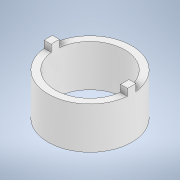
# Autodesk Inventor part: upperBase1
Saved by Autodesk Inventor 2021 (Build 250183000, 183)
## iProperties
Created: 2021-01-06
Part Number: upperBase1
Material: Generic
Document SubType Name: Modeling
Designer: awitc
Density: 1 g/cm^3
Appearance: Smooth - White
Author: awitc
Autodesk Inventor part; units mm, degrees
ref_plane "YZ Plane" through (0, 0, 0) normal (1, 0, 0) x (0, 1, 0)
ref_plane "XZ Plane" through (0, 0, 0) normal (0, 1, 0) x (-1, 0, 0)
ref_plane "XY Plane" through (0, 0, 0) normal (0, 0, 1) x (1, 0, 0)
sketch "Sketch1" plane through (0, 0, 0) normal (0, 1, 0) x (-1, 0, 0)
  line L0 (0, 0) -> (50, 0) construction
  line L1 (0, 0) -> (50, 0) construction
  line L2 (0, 0) -> (-36, 0)
  circle A0 centre (0, 0) radius 25
  line L3 (-60, -10) -> (-60, 10)
  circle A1 centre (0, 0) radius 61
  point P0 (62.509, -33.0548)
  point P1 (12.6591, 21.558)
  point P2 (24.4148, 5.3777)
  point P3 (24.4148, -5.3777)
  point P4 (-22.9129, 10)
  point P5 (-22.9129, -10)
  point P6 (12.6591, -21.558)
  dimension "d2" = 36
  dimension "d3" = 50
  dimension "d26" = 122
  constraints: 8 end point, 6 point on circle, 3 horizontal, 2 centre point, 2 coincident
  measures "d2" distance of L2.start L2.end
  measures "d3" diameter of A0
  measures "d26" diameter of A1
extrude "Extrusion1" add sketch "Sketch1" along normal blind 5 contours A0 | A1
sketch "Sketch2" plane through (0, 5, 0) normal (0, 1, 0) x (1, 0, 0)
  circle A0 centre (0, 0) radius 20
  dimension "d6" = 40
  constraints: 1 centre point, 1 coincident
  measures "d6" diameter of A0
extrude "Extrusion2" cut sketch "Sketch2" against normal up to next
sketch "Sketch3" plane through (0, 5, 0) normal (0, 1, 0) x (1, 0, 0)
  line L0 (22.1416, 4) -> (20.8701, 4)
  line L1 (22.1416, -4) -> (20.8701, -4)
  line L2 (24.6779, 4) -> (22.1416, 4)
  line L3 (24.6779, -4) -> (22.1416, -4)
  line L4 (-15.5618, -16.2506) -> (-14.5332, -15.5032)
  line L5 (-15.5618, 16.2506) -> (-14.5332, 15.5032)
  line L6 (-20.2641, -9.7784) -> (-19.2354, -9.0311)
  line L7 (-17.6137, -17.7414) -> (-15.5618, -16.2506)
  line L8 (-22.316, -11.2693) -> (-20.2641, -9.7784)
  line L9 (-20.2641, 9.7784) -> (-19.2354, 9.0311)
  line L10 (-17.6137, 17.7414) -> (-15.5618, 16.2506)
  line L11 (-22.316, 11.2693) -> (-20.2641, 9.7784)
  line L12 (-23.5374, 22.0452) -> (-13.679, 22.0452) construction
  arc A0 (-17.6137, -17.7414) -> (24.6779, -4) centre (0, 0) ccw
  arc A1 (24.6779, 4) -> (-17.6137, 17.7414) centre (0, 0) ccw
  arc A2 (-22.316, 11.2693) -> (-22.316, -11.2693) centre (0, 0) ccw
  line L13 (20.8701, 4) -> (15.8701, 4)
  line L14 (15.8701, 4) -> (15.8701, -4)
  line L15 (15.8701, -4) -> (20.8701, -4)
  line L16 (-14.5332, 15.5032) -> (-10.4881, 12.5643)
  line L17 (-10.4881, 12.5643) -> (-15.1903, 6.0922)
  line L18 (-15.1903, 6.0922) -> (-19.2354, 9.0311)
  line L19 (-19.2354, -9.0311) -> (-15.1903, -6.0922)
  line L20 (-15.1903, -6.0922) -> (-10.4881, -12.5643)
  line L21 (-10.4881, -12.5643) -> (-14.5332, -15.5032)
  circle A3 centre (-22.5, 0) radius 1.5
  circle A4 centre (0, 22.5) radius 1.5
  circle A5 centre (18.2029, 13.2252) radius 1.5
  circle A6 centre (18.2029, -13.2252) radius 1.5
  circle A7 centre (0, -22.5) radius 1.5
  circle A8 centre (0, 0) radius 4
  line L22 (0, 0) -> (8, 0)
  line L23 (8, 0) -> (8, 7.5)
  line L24 (8, 0) -> (8, -7.5)
  circle A9 centre (8, -7.5) radius 2.5
  circle A10 centre (8, 7.5) radius 2.5
  point P0 (-23.5374, -22.0452)
  point P1 (-28.2397, -15.5731)
  dimension "d9" = 36
  dimension "d10" = 5
  dimension "d11" = 5
  dimension "d12" = 3
  dimension "d13" = 3
  dimension "d14" = 3
  dimension "d15" = 3
  dimension "d16" = 3
  dimension "d17" = 8
  dimension "d18" = 8
  dimension "d19" = 7.5
  dimension "d20" = 7.5
  dimension "d21" = 5
  dimension "d22" = 5
  constraints: 50 end point, 11 centre point, 6 point on circle, 5 parallel, 4 coincident, 4 horizontal, 4 perpendicular, 2 vertical
  measures "d9" angle of L10 L12
  measures "d10" distance of L15.end L15.start
  measures "d11" distance of L16.start L17.start
  measures "d12" diameter of A3
  measures "d13" diameter of A4
  measures "d14" diameter of A5
  measures "d15" diameter of A6
  measures "d16" diameter of A7
  measures "d17" diameter of A8
  measures "d18" distance of L22.start L24.start
  measures "d19" distance of L24.start L23.end
  measures "d20" distance of L24.start L24.end
  measures "d21" diameter of A9
  measures "d22" diameter of A10
extrude "Extrusion3" cut sketch "Sketch3" against normal up to next contours A3 | A4 | A5 | A6 | A7
sketch "Sketch5" plane through (0, 5, 0) normal (0, 1, 0) x (1, 0, 0)
  line L0 (0, 0) -> (37.5601, 0) construction
  circle A0 centre (0, 0) radius 25
  line L1 (0, 0) -> (15.7675, -27.31)
  line L2 (0, 0) -> (31.5349, 0) construction
  line L3 (0, 0) -> (19.8269, 34.3411)
  line L4 (0, 0) -> (39.6537, 0) construction
  line L5 (12.5, 21.6506) -> (15, 25.9808)
  line L6 (12.5, -21.6506) -> (15, -25.9808)
  line L7 (15, -25.9808) -> (27.9904, -18.4808)
  line L8 (27.9904, -18.4808) -> (34.9904, -30.6051)
  line L9 (34.9904, -30.6051) -> (22, -38.1051)
  line L10 (22, -38.1051) -> (15, -25.9808)
  line L11 (22, -38.1051) -> (15, -25.9808)
  line L12 (15, -25.9808) -> (2.0096, -33.4808)
  line L13 (2.0096, -33.4808) -> (9.0096, -45.6051)
  line L14 (9.0096, -45.6051) -> (22, -38.1051)
  line L15 (15, 25.9808) -> (2.0096, 33.4808)
  line L16 (2.0096, 33.4808) -> (9.0096, 45.6051)
  line L17 (9.0096, 45.6051) -> (22, 38.1051)
  line L18 (22, 38.1051) -> (15, 25.9808)
  line L19 (22, 38.1051) -> (15, 25.9808)
  line L20 (15, 25.9808) -> (27.9904, 18.4808)
  line L21 (27.9904, 18.4808) -> (34.9904, 30.6051)
  line L22 (34.9904, 30.6051) -> (22, 38.1051)
  dimension "d41" = 50
  dimension "d47" = 60
  dimension "d48" = 60
  dimension "d49" = 5
  dimension "d50" = 5
  dimension "d51" = 15
  dimension "d52" = 14
  dimension "d53" = 15
  dimension "d54" = 15
  dimension "d55" = 14
  dimension "d56" = 15
  constraints: 46 end point, 11 equal length, 6 perpendicular, 4 point on line, 3 horizontal, 2 point on circle, 1 centre point, 1 coincident
  measures "d41" diameter of A0
  measures "d47" angle of L1 L2
  measures "d48" angle of L4 L3
  measures "d49" distance of L5.start L5.end
  measures "d50" distance of L6.start L6.end
  measures "d51" distance of L6.end L7.end
  measures "d52" distance of L7.end L8.end
  measures "d53" distance of L12.end L6.end
  measures "d54" distance of L5.end L15.end
  measures "d55" distance of L15.end L16.end
  measures "d56" distance of L20.end L5.end
extrude "Extrusion5" cut sketch "Sketch5" against normal up to next contours L7 L8 L9 L10 L1 | L1 L10 L14 L13 L12 | L15 L16 L17 L18 L3 | L3 L18 L22 L21 L20
sketch "Sketch6" plane through (0, 0, 0) normal (0, -1, 0) x (1, 0, 0)
  circle A0 centre (0, 0) radius 25
  circle A1 centre (0, 0) radius 28.75
  circle A2 centre (0, 0) radius 30
  dimension "d57" = 50
  dimension "d58" = 57.5
  constraints: 3 centre point, 3 coincident
  measures "d57" diameter of A0
  measures "d58" diameter of A1
extrude "Extrusion6" add sketch "Sketch6" along normal blind 30 contours A1 | A2
sketch "Sketch7" plane through (0, -30, 0) normal (0, -1, 0) x (1, 0, 0)
  circle A0 centre (26.875, 0) radius 1.5
  circle A1 centre (0, -26.875) radius 1.5
  circle A2 centre (-26.875, 0) radius 1.5
  circle A3 centre (0, 26.875) radius 1.5
  circle A4 centre (19.0035, 19.0035) radius 1.5
  circle A5 centre (19.0035, -19.0035) radius 1.5
  circle A6 centre (-19.0035, -19.0035) radius 1.5
  circle A7 centre (-19.0035, 19.0035) radius 1.5
  dimension "d62" = 3
  dimension "d63" = 3
  dimension "d64" = 3
  dimension "d65" = 3
  dimension "d67" = 3
  dimension "d68" = 3
  dimension "d69" = 3
  dimension "d70" = 3
  constraints: 8 centre point
  measures "d62" diameter of A0
  measures "d63" diameter of A1
  measures "d64" diameter of A2
  measures "d65" diameter of A3
  measures "d67" diameter of A4
  measures "d68" diameter of A5
  measures "d69" diameter of A6
  measures "d70" diameter of A7
extrude "Extrusion7" cut sketch "Sketch7" against normal blind 10
sketch "Sketch8" plane through (0, 0, 0) normal (0, -1, 0) x (1, 0, 0)
  line L0 (-37.9479, -22.6265) -> (-41.4746, -17.7724)
  line L1 (-47.9467, -22.4747) -> (-44.42, -27.3288)
  line L2 (-31.2231, -27.6292) -> (-27.6611, -32.4577)
  circle A0 centre (-42.9473, -22.5506) radius 1.5
  circle A1 centre (-26.2405, -27.6816) radius 1.5
  line L3 (-29.7189, 33.9527) -> (-36.191, 38.655)
  line L4 (-39.7177, 33.8009) -> (-33.2456, 29.0986)
  line L5 (-29.4532, 16.4547) -> (-35.9253, 21.157)
  line L6 (41.5, 10) -> (33.5, 10)
  line L7 (33.5, 4) -> (41.5, 4)
  line L8 (44, -10) -> (52, -10)
  circle A2 centre (48, -7) radius 1.5
  circle A3 centre (37.5, 7) radius 1.5
  circle A4 centre (-34.7183, 33.8768) radius 1.5
  circle A5 centre (-34.4526, 16.3788) radius 1.5
  point P0 (0, 0)
  point P1 (0, 0)
  point P2 (-32.9799, 11.6006)
  point P3 (44, -4)
  dimension "d73" = 3
  dimension "d74" = 3
  dimension "d75" = 3
  dimension "d76" = 3
  dimension "d77" = 3
  constraints: 18 end point, 6 centre point
  measures "d73" diameter of A0
  measures "d74" diameter of A1
  measures "d75" diameter of A2
  measures "d76" diameter of A3
  measures "d77" diameter of A5
extrude "Extrusion8" cut sketch "Sketch8" against normal blind 5
sketch "Sketch9" plane through (0, 5, 0) normal (0, 1, 0) x (1, 0, 0)
  line L0 (2.0096, -33.4808) -> (27.9904, -18.4808) projected
  line L1 (9.0096, -45.6051) -> (2.0096, -33.4808)
  line L2 (2.0096, -33.4808) -> (-0.5885, -34.9808)
  line L3 (-0.5885, -34.9808) -> (6.4115, -47.1051)
  line L4 (6.4115, -47.1051) -> (9.0096, -45.6051)
  line L5 (2.0096, 33.4808) -> (9.0096, 45.6051) projected
  line L6 (2.0096, 33.4808) -> (9.0096, 45.6051)
  line L7 (9.0096, 45.6051) -> (6.4115, 47.1051)
  line L8 (6.4115, 47.1051) -> (-0.5885, 34.9808)
  line L9 (-0.5885, 34.9808) -> (2.0096, 33.4808)
  point P0 (0, 0)
  dimension "d80" = 3
  dimension "d81" = 3
  constraints: 16 end point, 4 parallel, 3 perpendicular, 1 point on line
  measures "d80" distance of L2.end L0.start
  measures "d81" distance of L7.end L6.end
extrude "Extrusion9" cut sketch "Sketch9" against normal blind 10
sketch "Sketch10" plane through (0, 0, 0) normal (0, -1, 0) x (1, 0, 0)
  line L0 (6.4115, 47.1051) -> (-9.1769, 56.1051)
  line L1 (-9.1769, 56.1051) -> (-16.1769, 43.9808)
  line L2 (-16.1769, 43.9808) -> (-0.5885, 34.9808)
  line L3 (-9.1769, 56.1051) -> (-11.1769, 52.641)
  line L4 (-16.1769, 43.9808) -> (-14.1769, 47.4449)
  line L5 (-0.5885, 34.9808) -> (1.4115, 38.4449)
  line L6 (1.4115, 38.4449) -> (-2.0526, 40.4449)
  line L7 (6.4115, 47.1051) -> (4.4115, 43.641)
  line L8 (-0.5885, 34.9808) -> (6.4115, 47.1051) projected
  line L9 (4.4115, 43.641) -> (0.9474, 45.641)
  line L10 (27.9904, -18.4808) -> (-0.5885, -34.9808) projected
  line L11 (-16.1769, -43.9808) -> (-9.1769, -56.1051)
  line L12 (6.4115, -47.1051) -> (-0.5885, -34.9808)
  line L13 (-16.1769, -43.9808) -> (-14.1769, -47.4449)
  line L14 (-14.1769, -47.4449) -> (-10.7128, -45.4449)
  line L15 (-9.1769, -56.1051) -> (-11.1769, -52.641)
  line L16 (6.4115, -47.1051) -> (4.4115, -43.641)
  line L17 (-0.5885, -34.9808) -> (6.4115, -47.1051) projected
  line L18 (-0.5885, -34.9808) -> (1.4115, -38.4449)
  line L19 (6.4115, 47.1051) -> (3.8135, 48.6051)
  line L20 (3.8135, 48.6051) -> (-3.1865, 36.4808)
  line L21 (3.8135, 48.6051) -> (-2.6817, 52.3551)
  line L22 (1.8135, 45.141) -> (-2.0836, 47.391)
  line L23 (-2.0836, 47.391) -> (-5.0836, 42.1949)
  line L24 (-0.5885, -34.9808) -> (1.4115, -38.4449)
  line L25 (6.4115, -47.1051) -> (4.4115, -43.641)
  circle A0 centre (-5.5836, -41.3288) radius 1.5
  circle A1 centre (-1.5836, -48.257) radius 1.5
  line L26 (-2.0836, 47.391) -> (-1.5836, 48.257)
  line L27 (-5.0836, 42.1949) -> (-5.5836, 41.3288)
  circle A2 centre (-1.5836, 48.257) radius 1.5
  circle A3 centre (-5.5836, 41.3288) radius 1.5
  point P0 (0, 0)
  dimension "d85" = 14
  dimension "d86" = 4
  dimension "d88" = 4
  dimension "d92" = 4
  dimension "d93" = 4
  dimension "d94" = 4
  dimension "d95" = 4
  dimension "d98" = 18
  dimension "d99" = 4
  dimension "d101" = 4
  dimension "d103" = 4
  dimension "d129" = 3
  dimension "d130" = 7.5
  dimension "d137" = 4.5
  dimension "d140" = 4
  dimension "d146" = 3
  dimension "d148" = 1
  dimension "d149" = 1
  dimension "d150" = 3
  dimension "d151" = 3
  constraints: 50 end point, 14 point on line, 6 perpendicular, 4 centre point, 4 coincident, 1 collinear
  measures "d85" distance of L0.end L1.end
  measures "d86" distance of L0.end L3.end
  measures "d88" distance of L1.end L4.end
  measures "d92" distance of L2.end L5.end
  measures "d93" distance of L5.end L6.end
  measures "d94" distance of L0.start L7.end
  measures "d95" distance of L7.end L9.end
  measures "d98" distance of L10.end L11.start
  measures "d99" distance of L11.start L13.end
  measures "d101" distance of L11.end L15.end
  measures "d103" distance of L12.start L16.end
  measures "d129" distance of L0.start L19.end
  measures "d130" distance of L19.end L21.end
  measures "d137" distance of L22.start L22.end
  measures "d140" distance of L10.end L18.end
  measures "d146" diameter of A0
  measures "d148" distance of L23.start L26.end
  measures "d149" distance of L27.start L27.end
  measures "d150" diameter of A2
  measures "d151" diameter of A3
extrude "Extrusion13" cut sketch "Sketch10" against normal blind 10 contours A2 L23 L22 | L22 L23 A2 | A0 | A1 | A3
sketch "Sketch11" plane through (0, 5, 0) normal (0, 1, 0) x (1, 0, 0)
  circle A0 centre (0, 0) radius 61
  constraints: 1 centre point, 1 coincident
extrude "Extrusion14" cut sketch "Sketch11" against normal blind 5
sketch "Sketch12" plane through (0, 0, 0) normal (0, 1, 0) x (1, 0, 0)
  circle A0 centre (0, 0) radius 30
  circle A1 centre (0, 0) radius 30 projected
  circle A2 centre (0, 0) radius 25
  circle A3 centre (0, 0) radius 25 projected
  line L0 (-25, -3) -> (-29.8496, -3)
  line L1 (-24.8193, -3) -> (-25, -3)
  line L2 (-25, 3) -> (-24.8193, 3)
  line L3 (-29.8496, 3) -> (-24.8193, 3)
  line L4 (24.8193, -3) -> (29.8496, -3)
  line L5 (24.8193, 3) -> (29.8496, 3)
  constraints: 12 end point, 7 point on circle, 2 coincident, 2 collinear, 1 centre point, 1 horizontal, 1 parallel, 1 point on line, 3 other
extrude "Extrusion15" add sketch "Sketch12" along normal blind 5 contours A0 L4 A2 L5 | L3 L2 A2 L1 L0 A0
body "Solid1"
